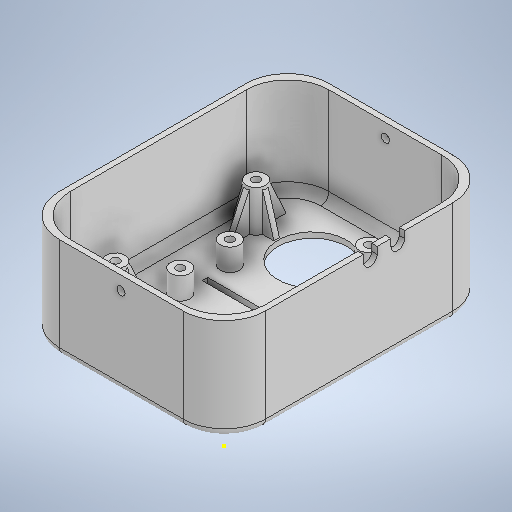
# Autodesk Inventor part: reduced_tortoise_2
Saved by Autodesk Inventor 2025.1 (Build 291241000, 241)
## iProperties
Created: 2025-04-14
Part Number: reduced_tortoise_2
Material: Generic
Document SubType Name: Modeling
Designer: Ian Ching
Density: 1 g/cm^3
Appearance: Default
Author: Ian Ching
Autodesk Inventor part; units mm, degrees
ref_plane "YZ Plane" through (0, 0, 0) normal (1, 0, 0) x (0, 1, 0)
ref_plane "XZ Plane" through (0, 0, 0) normal (0, 1, 0) x (-1, 0, 0)
ref_plane "XY Plane" through (0, 0, 0) normal (0, 0, 1) x (1, 0, 0)
sketch "Sketch1" plane through (0, 0, 0) normal (0, 1, 0) x (-1, 0, 0)
  line L0 (0, 0) -> (75, 0)
  line L1 (75, 0) -> (75, -98)
  line L2 (75, -98) -> (0, -98)
  line L3 (0, -98) -> (0, 0)
  dimension "d0" = 75
  dimension "d1" = 98
  constraints: 8 end point, 2 parallel, 1 horizontal, 1 perpendicular
  measures "d0" distance of L1.end L2.end
  measures "d1" distance of L0.end L1.end
extrude "Extrusion1" add sketch "Sketch1" along normal blind 2
sketch "Sketch2" plane through (0, 2, 0) normal (0, 1, 0) x (1, 0, 0)
  line L0 (-75, 98) -> (-75, 0) projected
  line L1 (0, 98) -> (-75, 98) projected
  line L2 (-75, 0) -> (0, 0)
  line L3 (0, 0) -> (0, 98)
  line L4 (0, 98) -> (-75, 98)
  line L5 (-75, 98) -> (-75, 0)
  line L6 (-37.5, 0) -> (-37.5, 98)
  line L7 (-73, 2) -> (-2, 2)
  line L8 (-2, 2) -> (-2, 96)
  line L9 (-2, 96) -> (-73, 96)
  line L10 (-73, 96) -> (-73, 2)
  line L11 (-37.5, 2) -> (-37.5, 96)
  point P0 (-37.5, 49)
  dimension "d4" = 71
  dimension "d5" = 94
  constraints: 20 end point, 6 midpoint, 4 parallel, 2 horizontal, 2 perpendicular
  measures "d4" distance of L9.end L8.end
  measures "d5" distance of L8.end L7.end
extrude "Extrusion2" add sketch "Sketch2" along normal blind 35 contours L1 L6 L9 L10 L7 L2 L0 | L1 L3 L2 L6 L7 L8 L9
sketch "Sketch3" plane through (0, 2, 0) normal (0, 1, 0) x (1, 0, 0)
  line L0 (-2, 2) -> (-73, 2) projected
  line L1 (-22, 23.5) -> (-63, 23.5)
  line L2 (-63, 23.5) -> (-63, 74.5)
  line L3 (-63, 74.5) -> (-22, 74.5)
  line L4 (-22, 74.5) -> (-22, 23.5)
  circle A0 centre (-42.5, 23.5) radius 12.5
  circle A1 centre (-42.5, 74.5) radius 12.5
  line L5 (-73, 2) -> (-73, 96) projected
  line L6 (-73, 49) -> (-2, 49)
  line L7 (-2, 96) -> (-2, 2) projected
  line L8 (-63, 49) -> (-73, 49)
  point P0 (0, 0)
  point P1 (0, 1)
  point P2 (-75, 1)
  dimension "d10" = 41
  dimension "d11" = 51
  dimension "d12" = 25
  dimension "d13" = 25
  dimension "d17" = 10
  constraints: 12 end point, 5 midpoint, 2 centre point, 2 parallel, 1 collinear, 1 horizontal, 1 perpendicular, 1 point on line, 1 other
  measures "d10" distance of L2.end L3.end
  measures "d11" distance of L1.end L2.end
  measures "d12" diameter of A0
  measures "d13" diameter of A1
  measures "d17" distance of L8.start L6.start
extrude "Extrusion3" cut sketch "Sketch3" against normal blind 40 contours A1 L3 | L3 A1 | A0 L1 | L1 A0
sketch "Sketch4" plane through (0, 2, 0) normal (0, 1, 0) x (1, 0, 0)
  line L0 (-73, 2) -> (-73, 96) projected
  line L1 (-73, 49) -> (-2, 49)
  line L2 (-2, 96) -> (-2, 2) projected
  line L3 (-63, 23.5) -> (-22, 23.5)
  line L4 (-22, 23.5) -> (-22, 74.5)
  line L5 (-22, 74.5) -> (-63, 74.5)
  line L6 (-63, 74.5) -> (-63, 23.5)
  circle A0 centre (-63, 23.5) radius 3.5
  circle A1 centre (-63, 74.5) radius 3.5
  circle A2 centre (-22, 23.5) radius 3.5
  circle A3 centre (-22, 74.5) radius 3.5
  line L7 (-73, 49) -> (-63, 49)
  point P0 (0, 0)
  dimension "d18" = 41
  dimension "d19" = 51
  dimension "d20" = 7
  dimension "d21" = 7
  dimension "d22" = 7
  dimension "d23" = 7
  dimension "d24" = 10
  constraints: 12 end point, 4 centre point, 4 coincident, 4 midpoint, 2 horizontal, 2 parallel, 1 perpendicular, 1 point on line
  measures "d18" distance of L5.end L4.end
  measures "d19" distance of L4.end L3.end
  measures "d20" diameter of A0
  measures "d21" diameter of A1
  measures "d22" diameter of A2
  measures "d23" diameter of A3
  measures "d24" distance of L7.end L7.start
extrude "Extrusion4" add sketch "Sketch4" along normal blind 15 contours A1 L5 L6 | L6 L5 A1 | A0 L3 L6 | L6 L3 A0 | A2 L3 L4 | L4 L3 A2 | A3 L5 L4 | L4 L5 A3
sketch "Sketch5" plane through (-63, 17, -23.5) normal (0, 1, 0) x (1, 0, 0)
  circle A0 centre (0, 0) radius 3.5 projected
  circle A1 centre (0, 0) radius 1.5
  circle A2 centre (0, 51) radius 3.5 projected
  circle A3 centre (0, 51) radius 1.5
  circle A4 centre (41, 51) radius 3.5 projected
  circle A5 centre (41, 51) radius 1.5
  circle A6 centre (41, 0) radius 3.5 projected
  circle A7 centre (41, 0) radius 1.5
  point P0 (63, -23.5)
  dimension "d27" = 3
  dimension "d28" = 3
  dimension "d29" = 3
  dimension "d30" = 3
  constraints: 4 centre point, 4 coincident
  measures "d27" diameter of A1
  measures "d28" diameter of A3
  measures "d29" diameter of A5
  measures "d30" diameter of A7
extrude "Extrusion5" cut sketch "Sketch5" against normal blind 10 contours A1 | A3 | A5 | A7
sketch "Sketch7" plane through (0, 2, 0) normal (0, 1, 0) x (1, 0, 0)
  line L0 (-23, 58) -> (-56, 58)
  line L1 (-56, 58) -> (-56, 40)
  line L2 (-56, 40) -> (-23, 40)
  line L3 (-23, 40) -> (-23, 58)
  line L4 (-2, 2) -> (-2, 96) projected
  line L5 (-73, 96) -> (-73, 2) projected
  circle A0 centre (-23, 58) radius 3.5
  circle A1 centre (-23, 40) radius 3.5
  circle A2 centre (-56, 58) radius 3.5
  circle A3 centre (-56, 40) radius 3.5
  circle A4 centre (-42.5, 74.5) radius 12.5 projected
  circle A5 centre (-42.5, 23.5) radius 12.5 projected
  line L6 (-42.5, 74.5) -> (-42.5, 23.5)
  line L7 (-42.5, -5.9281) -> (-42.5, 103.9281)
  line L8 (-56, 48) -> (-29, 48)
  line L9 (-29, 48) -> (-29, 50)
  line L10 (-29, 50) -> (-56, 50)
  line L11 (-56, 50) -> (-56, 48)
  line L12 (-56, 49) -> (-29, 49)
  point P0 (0, 0)
  point P1 (-37.5188, -25.1241)
  point P2 (-42.5, 49)
  dimension "d85" = 33
  dimension "d86" = 18
  dimension "d87" = 7
  dimension "d88" = 7
  dimension "d89" = 7
  dimension "d90" = 7
  dimension "d149" = 27
  dimension "d150" = 2
  constraints: 22 end point, 6 midpoint, 4 centre point, 4 coincident, 4 parallel, 2 horizontal, 2 perpendicular, 1 vertical
  measures "d85" distance of L2.end L1.end
  measures "d86" distance of L1.end L0.end
  measures "d87" diameter of A0
  measures "d88" diameter of A1
  measures "d89" diameter of A2
  measures "d90" diameter of A3
  measures "d149" distance of L10.end L9.end
  measures "d150" distance of L9.end L8.end
extrude "Extrusion7" add sketch "Sketch7" along normal blind 8 contours A2 L1 L0 | L0 L1 A2 | A0 L3 L0 | L0 L3 A0 | A1 L2 L3 | L3 L2 A1 | A3 L2 L1 | L1 L2 A3
sketch "Sketch8" plane through (-23, 10, -58) normal (0, 1, 0) x (1, 0, 0)
  circle A0 centre (0, 0) radius 3.5 projected
  circle A1 centre (0, 0) radius 1.5
  circle A2 centre (0, -18) radius 3.5 projected
  circle A3 centre (0, -18) radius 1.5
  circle A4 centre (-33, 0) radius 3.5 projected
  circle A5 centre (-33, 0) radius 1.5
  circle A6 centre (-33, -18) radius 3.5 projected
  circle A7 centre (-33, -18) radius 1.5
  point P0 (23, -58)
  dimension "d93" = 3
  dimension "d94" = 3
  dimension "d95" = 3
  dimension "d96" = 3
  constraints: 4 centre point, 4 coincident
  measures "d93" diameter of A1
  measures "d94" diameter of A3
  measures "d95" diameter of A5
  measures "d96" diameter of A7
extrude "Extrusion8" cut sketch "Sketch8" against normal blind 5 contours A1 | A3 | A5 | A7
sketch "Sketch9" plane through (0, 2, 0) normal (0, 1, 0) x (1, 0, 0)
  circle A0 centre (-23, 58) radius 1.5 projected
  circle A1 centre (-56, 40) radius 1.5 projected
  line L0 (-23, 58) -> (-56, 58)
  line L1 (-56, 58) -> (-56, 40)
  line L2 (-56, 40) -> (-23, 40)
  line L3 (-23, 40) -> (-23, 58)
  line L4 (-56, 48) -> (-29, 48)
  line L5 (-29, 48) -> (-29, 50)
  line L6 (-29, 50) -> (-56, 50)
  line L7 (-56, 50) -> (-56, 48)
  point P0 (0, 0)
  point P1 (-56, 49)
  point P2 (-56, 48)
  dimension "d145" = 27
  dimension "d146" = 2
  constraints: 16 end point, 4 parallel, 2 horizontal, 2 midpoint, 2 perpendicular
  measures "d145" distance of L6.end L5.end
  measures "d146" distance of L5.end L4.end
extrude "Extrusion9" cut sketch "Sketch9" against normal blind 5 contours L6 L5 L4 L1
sketch "Sketch10" plane through (0, 2, 0) normal (0, 1, 0) x (1, 0, 0)
  circle A0 centre (-22, 23.5) radius 1.5 projected
  circle A1 centre (-22, 23.5) radius 3.5
  line L0 (-2, 2) -> (-2, 96) projected
  line L1 (-2, 49) -> (-73, 49)
  line L2 (-73, 96) -> (-73, 2) projected
  circle A2 centre (-42.5, 74.5) radius 12.5 projected
  circle A3 centre (-42.5, 23.5) radius 12.5 projected
  line L3 (-42.5, 74.5) -> (-42.5, 23.5)
  line L4 (-14.5, 24.5) -> (-29.5, 24.5)
  line L5 (-29.5, 24.5) -> (-29.5, 22.5)
  line L6 (-29.5, 22.5) -> (-14.5, 22.5)
  line L7 (-14.5, 22.5) -> (-14.5, 24.5)
  line L8 (-23, 33.5) -> (-21, 33.5)
  line L9 (-21, 33.5) -> (-21, 13.5)
  line L10 (-21, 13.5) -> (-23, 13.5)
  line L11 (-23, 13.5) -> (-23, 33.5)
  line L12 (-22, 33.5) -> (-22, 13.5)
  line L13 (-14.5, 23.5) -> (-29.5, 23.5)
  circle A4 centre (-22, 74.5) radius 3.5
  line L14 (-14.5, 73.5) -> (-29.5, 73.5)
  line L15 (-29.5, 73.5) -> (-29.5, 75.5)
  line L16 (-29.5, 75.5) -> (-14.5, 75.5)
  line L17 (-14.5, 75.5) -> (-14.5, 73.5)
  line L18 (-23, 64.5) -> (-21, 64.5)
  line L19 (-21, 64.5) -> (-21, 84.5)
  line L20 (-21, 84.5) -> (-23, 84.5)
  line L21 (-23, 84.5) -> (-23, 64.5)
  circle A5 centre (-63, 23.5) radius 3.5
  line L22 (-70.5, 24.5) -> (-55.5, 24.5)
  line L23 (-55.5, 24.5) -> (-55.5, 22.5)
  line L24 (-55.5, 22.5) -> (-70.5, 22.5)
  line L25 (-70.5, 22.5) -> (-70.5, 24.5)
  line L26 (-62, 33.5) -> (-64, 33.5)
  line L27 (-64, 33.5) -> (-64, 13.5)
  line L28 (-64, 13.5) -> (-62, 13.5)
  line L29 (-62, 13.5) -> (-62, 33.5)
  line L30 (-70.5, 73.5) -> (-55.5, 73.5)
  line L31 (-55.5, 75.5) -> (-70.5, 75.5)
  line L32 (-70.5, 75.5) -> (-70.5, 73.5)
  line L33 (-55.5, 73.5) -> (-55.5, 75.5)
  circle A6 centre (-63, 74.5) radius 3.5
  line L34 (-62, 84.5) -> (-62, 64.5)
  line L35 (-64, 64.5) -> (-64, 84.5)
  line L36 (-64, 84.5) -> (-62, 84.5)
  line L37 (-62, 64.5) -> (-64, 64.5)
  point P0 (0, 0)
  point P1 (-23, 20.1459)
  point P2 (-21, 20.1459)
  point P3 (-18.6459, 22.5)
  point P4 (-18.6459, 24.5)
  point P5 (-23, 26.8541)
  point P6 (-21, 26.8541)
  point P7 (-25.3541, 22.5)
  point P8 (-25.3541, 24.5)
  point P9 (-66.3541, 22.5)
  point P10 (-66.3541, 24.5)
  point P11 (-62, 20.1459)
  point P12 (-64, 20.1459)
  point P13 (-59.6459, 24.5)
  point P14 (-59.6459, 22.5)
  point P15 (-64, 26.8541)
  point P16 (-62, 26.8541)
  point P17 (-64, 77.8541)
  point P18 (-62, 77.8541)
  point P19 (-62, 71.1459)
  point P20 (-64, 71.1459)
  point P21 (-66.3541, 73.5)
  point P22 (-66.3541, 75.5)
  point P23 (-59.6459, 75.5)
  point P24 (-59.6459, 73.5)
  point P25 (-25.3541, 73.5)
  point P26 (-25.3541, 75.5)
  point P27 (-21, 71.1459)
  point P28 (-23, 71.1459)
  point P29 (-18.6459, 75.5)
  point P30 (-18.6459, 73.5)
  point P31 (-23, 77.8541)
  point P32 (-21, 77.8541)
  point P33 (-20.3929, 71.3908)
  point P34 (-20.3929, 77.6092)
  point P35 (-20.3929, 20.3908)
  point P36 (-20.3929, 26.6092)
  dimension "d105" = 7
  dimension "d106" = 15
  dimension "d107" = 2
  dimension "d108" = 2
  dimension "d109" = 20
  constraints: 72 end point, 27 symmetric about line, 8 midpoint, 4 centre point, 4 parallel, 2 coincident, 2 horizontal, 2 perpendicular, 1 vertical, 5 other
  measures "d105" diameter of A1
  measures "d106" distance of L6.end L5.end
  measures "d107" distance of L5.end L4.end
  measures "d108" distance of L9.end L10.end
  measures "d109" distance of L8.end L9.end
extrude "Extrusion10" add sketch "Sketch10" along normal blind 14 contours L13 L7 L6 A1 | A1 L4 L7 L13 | A1 L12 L8 L9 | L9 L10 L12 A1 | A1 L11 L8 L12 | L12 L10 L11 A1 | L13 L5 L4 A1 | A1 L6 L5 L13 | A4 L16 L17 L14 | A4 L21 L20 L19 | L19 L18 L21 A4 | A4 L14 L15 L16 | A5 L22 L23 L24 | A5 L27 L26 L29 | L29 L28 L27 A5 | A5 L24 L25 L22 | L32 L31 A6 L30 | A6 L34 L37 L35 | L35 L36 L34 A6 | A6 L31 L33 L30
chamfer "Chamfer16" distance 6.6 distance2 14 2 edges at (-22, 16, -33.5) (-22, 16, -13.5) measured on face at (-22, 16, -33) measured on face at (-22, 16, -14)
chamfer "Chamfer17" distance 6.6 distance2 14 2 edges at (-22, 16, -64.5) (-22, 16, -84.5) measured on face at (-22, 16, -84) measured on face at (-22, 16, -65)
chamfer "Chamfer18" distance 6.6 distance2 14 2 edges at (-63, 16, -64.5) (-63, 16, -84.5) measured on face at (-63, 16, -65) measured on face at (-63, 16, -84)
chamfer "Chamfer19" distance 6.6 distance2 14 2 edges at (-63, 16, -13.5) (-63, 16, -33.5) measured on face at (-63, 16, -14) measured on face at (-63, 16, -33)
chamfer "Chamfer20" distance 4.1 distance2 14 2 edges at (-29.5, 16, -74.5) (-14.5, 16, -74.5) measured on face at (-15, 16, -74.5) measured on face at (-29, 16, -74.5)
chamfer "Chamfer21" distance 4.1 distance2 14 2 edges at (-29.5, 16, -23.5) (-14.5, 16, -23.5) measured on face at (-29, 16, -23.5) measured on face at (-15, 16, -23.5)
chamfer "Chamfer22" distance 4.1 distance2 14 2 edges at (-70.5, 16, -74.5) (-55.5, 16, -74.5) measured on face at (-56, 16, -74.5) measured on face at (-70, 16, -74.5)
chamfer "Chamfer23" distance 4.1 distance2 14 2 edges at (-70.5, 16, -23.5) (-55.5, 16, -23.5) measured on face at (-56, 16, -23.5) measured on face at (-70, 16, -23.5)
fillet "Fillet1" radius 15 8 edges at (-2, 19.5, -96) (0, 18.5, 0) (-75, 18.5, 0) (-75, 18.5, -98) (-73, 19.5, -96) (-2, 19.5, -2) (-73, 19.5, -2) (0, 18.5, -98)
sketch "Sketch12" plane through (0, 0, -15) normal (1, 0, 0) x (0, 0, -1)
  circle A0 centre (48, 34.5) radius 2.5
  circle A1 centre (38, 34.5) radius 2.5
  line L0 (68, 0) -> (68, 37) projected
  line L1 (68, 37) -> (48, 37)
  line L2 (48, 37) -> (48, 34.5)
  line L3 (48, 34.5) -> (68, 34.5)
  line L4 (68, 34.5) -> (68, 37)
  line L5 (68, 37) -> (38, 37)
  line L6 (38, 37) -> (38, 34.5)
  line L7 (38, 34.5) -> (68, 34.5)
  line L8 (68, 34.5) -> (68, 37)
  line L9 (50.5, 34.5) -> (50.5, 37)
  line L10 (45.5, 34.5) -> (45.5, 37)
  line L11 (40.5, 34.5) -> (40.5, 37)
  line L12 (35.5, 34.5) -> (35.5, 37)
  line L13 (66, 37) -> (2, 37) projected
  point P0 (-15, 0)
  dimension "d137" = 5
  dimension "d138" = 5
  dimension "d139" = 20
  dimension "d140" = 2.5
  dimension "d141" = 30
  dimension "d142" = 2.5
  constraints: 24 end point, 8 point on line, 4 parallel, 4 point on circle, 3 perpendicular, 3 tangent, 2 centre point, 2 coincident, 2 horizontal, 1 vertical, 2 other
  measures "d137" diameter of A0
  measures "d138" diameter of A1
  measures "d139" distance of L3.end L2.end
  measures "d140" distance of L2.end L1.end
  measures "d141" distance of L7.end L6.end
  measures "d142" distance of L6.end L5.end
extrude "Extrusion11" cut sketch "Sketch12" against normal blind 4 contours L3 L2 A0 | A0 L7 L3 | A0 L1 L9 | L2 L7 A0 | A0 L10 L5 | L7 L6 A1 | A1 L6 L7 | A1 L5 L11 | A1 L12 L13
fillet "Face Fillet1" radius 3 1 edges at (-68.6066, 2, -6.3934)
fillet "Face Fillet2" radius 3 1 edges at (0, 0, -49)
sketch "Sketch16" plane through (-60, 37, 0) normal (0, 0, 1) x (1, 0, 0)
  line L0 (45, 0) -> (0, 0) projected
  line L1 (0, 0) -> (45, 0)
  line L2 (45, 0) -> (45, -5)
  line L3 (45, -5) -> (0, -5)
  line L4 (0, -5) -> (0, 0)
  circle A0 centre (22.5, -5) radius 1.5
  point P0 (60, -37)
  dimension "d164" = 45
  dimension "d165" = 5
  dimension "d166" = 3
  constraints: 8 end point, 2 parallel, 1 centre point, 1 horizontal, 1 midpoint, 1 perpendicular
  measures "d164" distance of L2.end L3.end
  measures "d165" distance of L1.end L2.end
  measures "d166" diameter of A0
extrude "Extrusion13" cut sketch "Sketch16" against normal blind 98 contours A0 L3 | L3 A0
sketch "Sketch17" plane through (0, 2, 0) normal (0, 1, 0) x (1, 0, 0)
  point P0 (0, 0)
body "Solid1"
